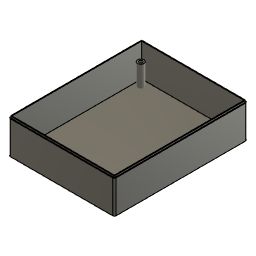
Base da Case (Autodesk Fusion 360 design; units mm, degrees)
Autodesk Fusion 360 part; units mm, degrees
sketch "Sketch1" plane through (0, 0, 0) normal (0, 1, 0) x (1, 0, 0)
  line L0 (0, 0) -> (66, 0)
  line L1 (66, 0) -> (66, -83)
  line L2 (66, -83) -> (0, -83)
  line L3 (0, -83) -> (0, 0)
  circle A0 centre (4.286, -4.8) radius 2
  circle A1 centre (4.286, -4.8) radius 1
  circle A2 centre (61.36, -4.8) radius 2
  circle A3 centre (61.36, -4.8) radius 1
  circle A4 centre (4.286, -78.46) radius 2
  circle A5 centre (4.286, -78.46) radius 1
  circle A6 centre (61.36, -78.46) radius 2
  circle A7 centre (61.36, -78.46) radius 1
  line L4 (65, -82) -> (1, -82)
  line L5 (1, -82) -> (1, -1)
  line L6 (1, -1) -> (65, -1)
  line L7 (65, -1) -> (65, -82)
  dimension "d1" = 66
  dimension "d2" = 83
  dimension "d5" = 4
  dimension "d6" = 2
  dimension "d8" = 4
  dimension "d9" = 2
  dimension "d11" = 4
  dimension "d12" = 2
  dimension "d14" = 4
  dimension "d15" = 2
  dimension "d16" = 1
  constraint horizontal L0
  constraint vertical L1
  constraint horizontal L2
  constraint vertical L3
  constraint coincident L0.start L3.end
  constraint concentric A0 A1
  constraint concentric A2 A3
  constraint concentric A4 A5
  constraint concentric A6 A7
  measures "d1" distance of L0.start L0.end
  measures "d2" distance of L0.start L2.end
  measures "d5" diameter of A0
  measures "d6" diameter of A1
  measures "d8" diameter of A2
  measures "d9" diameter of A3
  measures "d11" diameter of A4
  measures "d12" diameter of A5
  measures "d14" diameter of A6
  measures "d15" diameter of A7
extrude "Extrude1" add sketch "Sketch1" along normal blind 21.5 contours L0 L1 L2 L3 makes body 1
extrude "Extrude2" add sketch "Sketch1" along normal blind 1 contours A0 | A1 | A2 | A3 | A4 | A5 | A6 | A7 | L4 L5 L6 L7 bodies 1
extrude "Extrude3" add sketch "Sketch1" along normal blind 13.903 separate body contours A0 | A2 | A4 | A6 makes body 2 at (63.3501, 4.6343, 4.9991) makes body 3 at (2.443, 9.2687, 79.2369) makes body 4 at (6.2761, 4.6343, 4.9991) makes body 5 at (63.3203, 9.2687, 78.8563)
fillet "Fillet1" radius 1 4 edges at (0, 10.75, 0) (66, 10.75, 0) (66, 10.75, 83) (0, 10.75, 83) on bodies 1
sketch "Sketch2" plane through (0, 21.5, 0) normal (0, 1, 0) x (-1, 0, 0)
  arc A0 (0, 82) -> (-1, 83) centre (-1, 82) ccw
  line L0 (-1, 83) -> (-65, 83)
  arc A1 (-65, 83) -> (-66, 82) centre (-65, 82) ccw
  line L1 (-66, 82) -> (-66, 1)
  arc A2 (-66, 1) -> (-65, 0) centre (-65, 1) ccw
  line L2 (-65, 0) -> (-1, 0)
  arc A3 (-1, 0) -> (0, 1) centre (-1, 1) ccw
  line L3 (0, 1) -> (0, 82)
  line L4 (-1, 1) -> (-65, 1)
  line L5 (-65, 1) -> (-65, 82)
  line L6 (-65, 82) -> (-1, 82)
  line L7 (-1, 82) -> (-1, 1)
  arc A4 (-65, 82.5) -> (-65.5, 82) centre (-65, 82) ccw
  line L8 (-65.5, 82) -> (-65.5, 1)
  arc A5 (-65.5, 1) -> (-65, 0.5) centre (-65, 1) ccw
  line L9 (-65, 0.5) -> (-1, 0.5)
  arc A6 (-1, 0.5) -> (-0.5, 1) centre (-1, 1) ccw
  line L10 (-0.5, 1) -> (-0.5, 82)
  arc A7 (-0.5, 82) -> (-1, 82.5) centre (-1, 82) ccw
  line L11 (-1, 82.5) -> (-65, 82.5)
  dimension "d25" = -0.5
extrude "Extrude4" cut sketch "Sketch2" against normal blind 1 contours A0 L0 A1 L1 A2 L2 A3 L3 bodies 1
